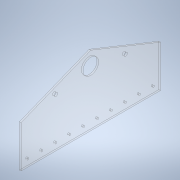
# Autodesk Inventor part: Jeep Plate
Saved by Autodesk Inventor 2020 (Build 240168000, 168)
## iProperties
Created: 2020-02-06
Part Number: Jeep Plate
Material: Polycarbonate, Clear
Document SubType Name: Modeling
Designer: aidan
Density: 1.2 g/cm^3
Appearance: Polycarbonate - Clear
Author: aidan
Autodesk Inventor part; units mm, degrees
ref_plane "YZ Plane" through (0, 0, 0) normal (1, 0, 0) x (0, 1, 0)
ref_plane "XZ Plane" through (0, 0, 0) normal (0, 1, 0) x (-1, 0, 0)
ref_plane "XY Plane" through (0, 0, 0) normal (0, 0, 1) x (1, 0, 0)
sketch "Sketch1" plane through (0, 0, 0) normal (1, 0, 0) x (0, 1, 0)
  line L0 (23.1056, 132.8959) -> (-53.0944, 132.8959)
  line L1 (-53.0944, 132.8959) -> (-53.0944, -121.1041)
  line L2 (-53.0944, -121.1041) -> (23.1056, -121.1041)
  line L3 (23.1056, 132.8959) -> (73.9056, 5.8959)
  line L4 (73.9056, 5.8959) -> (23.1056, -121.1041)
  line L5 (73.9056, 5.8959) -> (-53.0944, 5.8959) construction
  point P0 (0, 0)
  dimension "d0" = 76.2
  dimension "d1" = 254
  constraints: 12 end point, 1 equal length, 1 horizontal, 1 midpoint, 1 parallel, 1 perpendicular
  measures "d0" distance of L0.start L0.end
  measures "d1" distance of L0.end L1.end
extrude "Extrusion1" add sketch "Sketch1" along normal blind 2.9972
sketch "Sketch2" plane through (2.9972, 0, 0) normal (1, 0, 0) x (0, 0, -1)
  circle A0 centre (-120.1959, -40.3944) radius 1.7272
  line L0 (-132.8959, 23.1056) -> (-132.8959, -53.0944) projected
  line L1 (-132.8959, -53.0944) -> (121.1041, -53.0944) projected
  point P0 (0, 0)
  dimension "d5" = 12.7
  dimension "d6" = 12.7
  dimension "d7" = 3.4544
  constraints: 1 centre point
  measures "d5" distance from line of L0 A0.centre
  measures "d6" distance from line of L1 A0.centre
  measures "d7" diameter of A0
extrude "Extrusion2" cut sketch "Sketch2" against normal through all
pattern_linear "Rectangular Pattern1" count 10 spacing 25.4 along (0, 0, -1) of "Extrusion2"
sketch "Sketch3" plane through (2.9972, 0, 0) normal (1, 0, 0) x (0, 0, -1)
  circle A0 centre (-5.8959, 48.5056) radius 14.2875
  line L0 (121.1041, 23.1056) -> (-5.8959, 73.9056) projected
  line L1 (-5.8959, 73.9056) -> (-5.8959, 48.5056) construction
  point P0 (0, 0)
  dimension "d13" = 28.575
  dimension "d14" = 25.4
  constraints: 2 end point, 1 centre point, 1 vertical
  measures "d13" diameter of A0
  measures "d14" distance of L1.end L0.end
extrude "Extrusion3" cut sketch "Sketch3" against normal through all
sketch "Sketch4" plane through (2.9972, 0, 0) normal (1, 0, 0) x (0, 0, -1)
  circle A0 centre (-69.3959, 35.8056) radius 3.175
  circle A1 centre (57.6041, 35.8056) radius 3.175
  line L0 (-69.3959, 35.8056) -> (57.6041, 35.8056) construction
  line L1 (121.1041, 23.1056) -> (-5.8959, 73.9056) projected
  line L2 (-5.8959, 73.9056) -> (-5.8959, 17.32) construction
  point P0 (0, 0)
  dimension "d17" = 6.35
  dimension "d18" = 127
  dimension "d19" = 63.5
  dimension "d20" = 38.1
  constraints: 4 end point, 2 centre point, 1 equal radius, 1 horizontal, 1 vertical
  measures "d17" diameter of A0
  measures "d18" distance of L0.start L0.end
  measures "d19" distance from line of L0.end L2
  measures "d20" distance from line of L0 L1.end
extrude "Extrusion4" cut sketch "Sketch4" against normal through all
body "Solid1"
